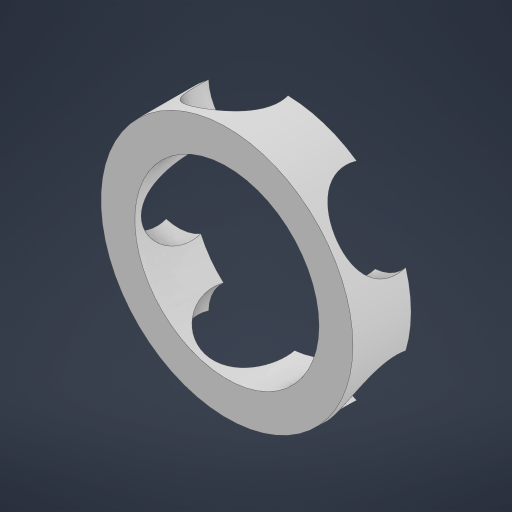
# Autodesk Inventor part: Hex Bearing Spacer
Saved by Autodesk Inventor 2023 (Build 270158000, 158)
## iProperties
Created: 2022-10-15
Part Number: Hex Bearing Spacer
Material: Generic
Document SubType Name: Modeling
Designer: izack
Density: 1 g/cm^3
Appearance: Default
Author: izack
Autodesk Inventor part; units mm, degrees
ref_plane "YZ Plane" through (0, 0, 0) normal (1, 0, 0) x (0, 1, 0)
ref_plane "XZ Plane" through (0, 0, 0) normal (0, 1, 0) x (-1, 0, 0)
ref_plane "XY Plane" through (0, 0, 0) normal (0, 0, 1) x (1, 0, 0)
sketch "Sketch1" plane through (0, 0, 0) normal (0, 0, 1) x (1, 0, 0)
  circle A0 centre (8.7, 0) radius 3.375
  circle A1 centre (8.7, 0) radius 6.5
  circle A2 centre (8.7, 0) radius 4.75
  point P0 (0, 0)
  dimension "d0" = 13
  dimension "d1" = 9.5
  constraints: 3 centre point, 2 coincident, 2 other
  measures "d0" diameter of A1
  measures "d1" diameter of A2
extrude "Extrusion1" add sketch "Sketch1" against normal blind 3 contours A1
ref_plane "Work Plane1" through (8.7, 0, -2.5) normal (0, 0, 1) x (1, 0, 0)
sketch "Sketch2" plane through (8.7, 0, -2.5) normal (0, 0, 1) x (1, 0, 0)
  circle A0 centre (0, 0) radius 6.5 projected
  circle A1 centre (0, 0) radius 4.75 projected
  circle A2 centre (0, 0) radius 5.5
  circle A3 centre (-5.5, 0) radius 2.3
  line L0 (-7.8, 0) -> (-3.2, 0)
  point P0 (-8.7, 0)
  dimension "d5" = 11
  dimension "d6" = 4.6
  constraints: 2 end point, 2 point on circle, 1 centre point, 1 coincident, 1 horizontal, 1 horizontal alignment, 2 other
  measures "d6" diameter of A3
revolve "Revolution1" cut sketch "Sketch2" angle 360 about axis through (0.9, 0, -2.5) along (1, 0, 0) picked at (-6.9008, -0.416) picked at (-5.7866, -1.7687) picked at (-5.232, -0.2566) picked at (-4.2335, -0.3826) contours A3 L0 A0 | A0 L0 A2 A3 | A2 L0 A1 A3 | A1 L0 A3
pattern_circular "Circular Pattern1" count 5 over 360 about axis through (8.7, 0, -3) along (0, 0, 1) of "Revolution1"
body "Solid1"
